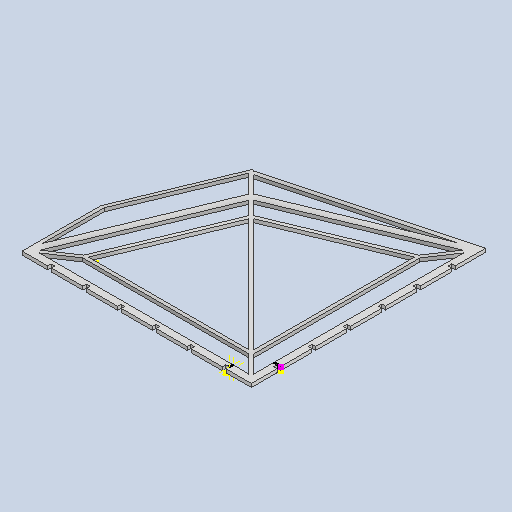
# Autodesk Inventor part: side_sail
Saved by Autodesk Inventor 2024 (Build 280153000, 153)
## iProperties
Created: 2024-04-09
Part Number: side_sail
Material: 一般
Document SubType Name: Modeling
Designer: USER
Density: 1 g/cm^3
Appearance: 預設
Author: USER
Autodesk Inventor part; units mm, degrees
ref_plane "YZ Plane" through (0, 0, 0) normal (1, 0, 0) x (0, 1, 0)
ref_plane "XZ Plane" through (0, 0, 0) normal (0, 1, 0) x (-1, 0, 0)
ref_plane "XY Plane" through (0, 0, 0) normal (0, 0, 1) x (1, 0, 0)
sketch "草圖1" plane through (0, 0, 0) normal (0, 1, 0) x (-1, 0, 0)
  line L0 (0, 0) -> (0, -200)
  line L1 (0, 0) -> (200, 0)
  line L2 (0, 0) -> (141.4214, -141.4214)
  line L3 (200, 0) -> (141.4214, -141.4214)
  line L4 (141.4214, -141.4214) -> (0, -200)
  line L5 (191.0204, -6) -> (6, -6)
  line L6 (6, -6) -> (6, -191.0204)
  line L7 (6, -191.0204) -> (136.8292, -136.8292)
  line L8 (136.8292, -136.8292) -> (191.0204, -6)
  line L9 (2.1213, 0) -> (142.0427, -139.9214)
  line L10 (0, -2.1213) -> (139.9214, -142.0427)
  line L11 (168.5713, -21) -> (21, -21)
  line L12 (21, -21) -> (21, -168.5713)
  line L13 (21, -168.5713) -> (125.3487, -125.3487)
  line L14 (125.3487, -125.3487) -> (168.5713, -21)
  line L15 (164.0815, -24) -> (24, -24)
  line L16 (24, -24) -> (24, -164.0815)
  line L17 (24, -164.0815) -> (123.0526, -123.0526)
  line L18 (123.0526, -123.0526) -> (164.0815, -24)
  line L19 (191.0204, -6) -> (168.5713, -21)
  line L20 (191.8537, -7.2472) -> (169.4046, -22.2472)
  line L21 (190.187, -4.7528) -> (167.7379, -19.7528)
  line L22 (167.7379, -19.7528) -> (161.3815, -24)
  line L23 (169.4046, -22.2472) -> (163.0482, -26.4944)
  line L24 (24, -164.0815) -> (6, -191.0204)
  line L25 (25.2472, -164.9148) -> (7.2472, -191.8537)
  line L26 (22.7528, -163.2481) -> (4.7528, -190.187)
  line L27 (175, 0) -> (171.8, 0)
  line L28 (171.8, 0) -> (171.8, -3)
  line L29 (171.8, -3) -> (175, -3)
  line L30 (175, -3) -> (175, 0)
  line L31 (141.8, -3) -> (145, -3)
  line L32 (141.8, 0) -> (141.8, -3)
  line L33 (145, -3) -> (145, 0)
  line L34 (111.8, -3) -> (115, -3)
  line L35 (111.8, 0) -> (111.8, -3)
  line L36 (115, -3) -> (115, 0)
  line L37 (81.8, -3) -> (85, -3)
  line L38 (81.8, 0) -> (81.8, -3)
  line L39 (85, -3) -> (85, 0)
  line L40 (51.8, -3) -> (55, -3)
  line L41 (51.8, 0) -> (51.8, -3)
  line L42 (55, -3) -> (55, 0)
  line L43 (21.8, -3) -> (25, -3)
  line L44 (21.8, 0) -> (21.8, -3)
  line L45 (25, -3) -> (25, 0)
  line L46 (0, -200) -> (0, -222)
  line L47 (0, -222) -> (156.9777, -156.9777)
  line L48 (200, 0) -> (222, 0)
  line L49 (141.4214, -141.4214) -> (156.9777, -156.9777)
  line L50 (222, 0) -> (156.9777, -156.9777)
  line L51 (197.0204, 0) -> (197.0204, -60.3062)
  line L52 (0, -222) -> (0, -225)
  line L53 (0, -225) -> (159.099, -159.099)
  line L54 (156.9777, -156.9777) -> (159.099, -159.099)
  line L55 (159.099, -159.099) -> (225, 0)
  line L56 (222, 0) -> (225, 0)
  line L57 (197.0204, -60.3062) -> (197.0204, -67.5488)
  line L58 (0, -200) -> (0, -222)
  line L59 (6, -197.5147) -> (6, -219.5147)
  line L60 (194.0204, -67.5488) -> (194.0204, -14.4361)
  line L61 (142.0427, -139.9214) -> (157.599, -155.4777)
  line L62 (139.9214, -142.0427) -> (157.599, -159.7203)
  line L63 (0, -22) -> (3, -22)
  line L64 (3, -22) -> (3, -25.2)
  line L65 (3, -25.2) -> (0, -25.2)
  line L66 (0, -25.2) -> (0, -22)
  line L67 (3, -52) -> (3, -55.2)
  line L68 (0, -52) -> (3, -52)
  line L69 (3, -55.2) -> (0, -55.2)
  line L70 (3, -82) -> (3, -85.2)
  line L71 (0, -82) -> (3, -82)
  line L72 (3, -85.2) -> (0, -85.2)
  line L73 (3, -112) -> (3, -115.2)
  line L74 (0, -112) -> (3, -112)
  line L75 (3, -115.2) -> (0, -115.2)
  line L76 (3, -142) -> (3, -145.2)
  line L77 (0, -142) -> (3, -142)
  line L78 (3, -145.2) -> (0, -145.2)
  line L79 (3, -172) -> (3, -175.2)
  line L80 (0, -172) -> (3, -172)
  line L81 (3, -175.2) -> (0, -175.2)
  line L82 (155.4777, -157.599) -> (6, -197.5147)
  line L83 (155.7761, -159.5894) -> (8, -199.0507)
  line L84 (8, -199.0507) -> (8, -219.5147)
  line L85 (155.0907, -156.1498) -> (4.5, -196.3627)
  line L86 (4.5, -196.3627) -> (4.5, -219.5147)
  line L87 (155.7761, -159.5894) -> (158.7857, -158.7857)
  line L88 (8, -199.0507) -> (0, -201.187)
  point P0 (8.1213, -6)
  point P1 (137.4505, -135.3292)
  point P2 (135.3292, -137.4505)
  point P3 (6, -8.1213)
  point P4 (121.5526, -123.6739)
  point P5 (24, -26.1213)
  point P6 (21, -23.1213)
  point P7 (123.8487, -125.97)
  point P8 (123.6739, -121.5526)
  point P9 (125.97, -123.8487)
  point P10 (23.1213, -21)
  point P11 (26.1213, -24)
  point P12 (21, -165.8714)
  point P13 (6, -188.3204)
  point P14 (8.4944, -189.9871)
  point P15 (23.4944, -167.5381)
  point P16 (188.3204, -6)
  point P17 (165.8714, -21)
  point P18 (167.5381, -23.4944)
  point P19 (189.9871, -8.4944)
  point P20 (171.8, 0)
  point P21 (141.8, 0)
  point P22 (111.8, 0)
  point P23 (81.8, 0)
  point P24 (51.8, 0)
  point P25 (21.8, 0)
  point P26 (156.9777, -156.9777)
  point P27 (197.0204, -7.1935)
  point P28 (157.5991, -156.7203)
  point P29 (0, -25.2)
  point P30 (0, -55.2)
  point P31 (0, -85.2)
  point P32 (0, -115.2)
  point P33 (0, -145.2)
  point P34 (0, -175.2)
  point P35 (154.2524, -156.3737)
  point P36 (16.5488, -193.1453)
  point P37 (157.1115, -159.2328)
  point P38 (0, -201.187)
  dimension "d0" = 200
  dimension "d1" = 200
  dimension "d2" = 45
  dimension "d3" = 67.5
  dimension "d4" = 6
  dimension "d5" = 1.5
  dimension "d6" = 1.5
  dimension "d9" = 15
  dimension "d10" = 3
  dimension "d11" = 1.5
  dimension "d12" = 1.5
  dimension "d13" = 1.5
  dimension "d14" = 1.5
  dimension "d15" = 3
  dimension "d16" = 3.2
  dimension "d17" = 25
  dimension "d20" = 30
  dimension "d27" = 22
  dimension "d28" = 22
  dimension "d29" = 6
  dimension "d30" = 3
  dimension "d31" = 3
  dimension "d32" = 6
  dimension "d34" = 3
  dimension "d35" = 3
  dimension "d36" = 3.2
  dimension "d37" = 22
  dimension "d40" = 30
  dimension "d49" = 2
  dimension "d50" = 1.5
  constraints: 178 end point, 22 point on line, 16 parallel, 7 collinear, 7 vertical, 6 horizontal, 2 perpendicular, 1 coincident, 81 other
  measures "d0" distance of L0.start L0.end
  measures "d1" distance of L0.start L1.end
  measures "d2" angle of L0 L2
  measures "d3" angle of L3 L1
  measures "d4" distance between parallel lines of L1 L5
  measures "d5" distance between parallel lines of L2 L9
  measures "d6" distance between parallel lines of L2 L10
  measures "d9" distance between parallel lines of L8 L14
  measures "d10" distance between parallel lines of L14 L18
  measures "d11" distance between parallel lines of L19 L20
  measures "d12" distance between parallel lines of L19 L21
  measures "d13" distance between parallel lines of L24 L25
  measures "d14" distance between parallel lines of L24 L26
  measures "d15" distance of L29.end L27.start
  measures "d16" distance of L28.end L29.end
  measures "d17" horizontal distance of L1.end L29.end
  measures "d20" distance of L28.end L31.start
  measures "d27" distance of L0.end L46.end
  measures "d28" distance of L1.end L48.end
  measures "d29" distance from line of L5.start L51
  measures "d30" distance of L46.end L52.end
  measures "d31" distance of L48.end L55.end
  measures "d32" distance between parallel lines of L46 L59
  measures "d34" distance between parallel lines of L60 L51
  measures "d35" distance of L64.end L65.end
  measures "d36" distance of L63.end L64.end
  measures "d37" distance of L0.start L63.start
  measures "d40" distance of L63.end L67.start
  measures "d49" distance between parallel lines of L82 L83
  measures "d50" distance between parallel lines of L82 L85
extrude "擠出1" add sketch "草圖1" along normal blind 3 contours L2 L6 L10 L0 | L1 L9 L5 L2 | L10 L6 L7 L4 L85 L86 L0 L81 L79 L80 L78 L76 L77 L75 L73 L74 L72 L70 L71 L69 L67 L68 L65 L64 L63 | L1 L44 L43 L45 L41 L40 L42 L38 L37 L39 L35 L34 L36 L32 L31 L33 L28 L29 L30 L51 L3 L9 L8 L5 | L5 L9 L11 L2 | L2 L12 L10 L6 | L11 L9 L15 L2 | L2 L16 L10 L12 | L26 L12 L24 L6 | L10 L16 L24 L12 | L5 L19 L11 L22 L21 | L11 L22 L15 L9 | L15 L9 L18 L2 | L2 L17 L10 L16 | L24 L13 L25 L7 | L8 L20 L23 L14 L19 | L11 L14 L23 L18 L15 L22 | L18 L9 L14 L2 | L2 L13 L10 L17 | L24 L17 L10 L13 | L18 L23 L14 L9 | L14 L9 L8 L2 | L2 L7 L10 L13 | L7 L2 L4 L10 | L9 L3 L2 L8 | L4 L49 L47 L62 | L61 L50 L49 L3 | L85 L62 L82 L4 | L4 L86 L85 | L3 L51 L50 L60 | L50 L57 L55 L54 | L54 L87 L62 L47 | L59 L88 L86 L4 | L82 L47 L83 L88 L59 | L62 L87 L83 L47 | L54 L53 L62 L87 | L86 L88 L46 L4
sketch "草圖2" plane through (-3, 0, -25.2) normal (0, 0, 1) x (1, 0, 0)
  line L0 (0, 0) -> (0, 3) projected
  line L1 (-154.599, 3) -> (-156.099, 3) projected
  line L2 (0, 0) -> (-3, 0)
  line L3 (-3, 0) -> (-3, 3)
  line L4 (-3, 3) -> (0, 3)
  line L5 (0, 3) -> (0, 0)
  circle A0 centre (-1.5, 1.5) radius 2.1213
  point P0 (3, 0)
  point P1 (3, 3)
  dimension "d45" = 3
  dimension "d46" = 4.2426
  constraints: 8 end point, 2 parallel, 2 point on circle, 1 centre point, 1 horizontal, 1 perpendicular, 1 point on line
  measures "d45" distance of L0.end L3.end
  measures "d46" diameter of A0
sketch "草圖3" plane through (-21.8, 0, -3) normal (-1, 0, 0) x (0, 0, 1)
  line L0 (0, 3) -> (-3, 3)
  line L1 (-3, 3) -> (-3, 0)
  line L2 (-3, 0) -> (0, 0)
  line L3 (0, 0) -> (0, 3)
  circle A0 centre (-1.5, 1.5) radius 2.1213
  point P0 (3, 0)
  dimension "d47" = 4.2426
  dimension "d48" = 1.5
  constraints: 8 end point, 2 parallel, 1 horizontal, 1 perpendicular, 3 other
  measures "d48" distance from line of point (-1.5, 1.5) L3
